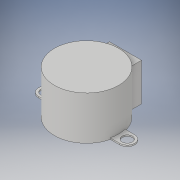
# Autodesk Inventor part: PasAPasCarcasse
Saved by Autodesk Inventor 2019 (Build 230136000, 136)
## iProperties
Created: 2020-12-11
Part Number: PasAPasCarcasse
Material: Générique
Document SubType Name: Modeling
Designer: tom.mousset
Density: 1 g/cm^3
Appearance: Par défaut
Author: tom.mousset
Autodesk Inventor part; units mm, degrees
ref_plane "YZ Plane" through (0, 0, 0) normal (1, 0, 0) x (0, 1, 0)
ref_plane "XZ Plane" through (0, 0, 0) normal (0, 1, 0) x (-1, 0, 0)
ref_plane "XY Plane" through (0, 0, 0) normal (0, 0, 1) x (1, 0, 0)
sketch "Esquisse1" plane through (0, 0, 0) normal (0, 1, 0) x (-1, 0, 0)
  circle A0 centre (0, 0) radius 14
  dimension "d0" = 28
  constraints: 1 centre point, 1 coincident
  measures "d0" diameter of A0
extrude "Extrusion1" add sketch "Esquisse1" along normal blind 19
sketch "Esquisse2" plane through (0, 0, 0) normal (0, -1, 0) x (1, 0, 0)
  line L0 (-21, -3.25) -> (21, -3.25)
  line L1 (21, -3.25) -> (21, 3.25)
  line L2 (21, 3.25) -> (-21, 3.25)
  line L3 (-21, 3.25) -> (-21, -3.25)
  line L4 (-21, -3.25) -> (21, 3.25) construction
  line L5 (21, -3.25) -> (-21, 3.25) construction
  circle A0 centre (-17.75, 0) radius 2.25
  circle A1 centre (17.75, 0) radius 2.25
  arc A2 (-17.75, 3.25) -> (-17.75, -3.25) centre (-17.75, 0) ccw
  arc A3 (17.75, -3.25) -> (17.75, 3.25) centre (17.75, 0) ccw
  circle A4 centre (0, 0) radius 14 projected
  arc A5 (13.6175, -3.25) -> (13.6175, 3.25) centre (0, 0) ccw
  arc A6 (-13.6175, 3.25) -> (-13.6175, -3.25) centre (0, 0) ccw
  line L6 (-17.75, 3.25) -> (-13.6175, 3.25)
  line L7 (-17.75, -3.25) -> (-13.6175, -3.25)
  line L8 (13.6175, -3.25) -> (17.75, -3.25)
  line L9 (17.75, 3.25) -> (13.6175, 3.25)
  dimension "d3" = 42
  dimension "d4" = 6.5
  dimension "d5" = 4.5
  dimension "d6" = 4.5
  dimension "d7" = 3.25
  dimension "d8" = 3.25
  constraints: 20 end point, 12 point on circle, 8 point on line, 6 centre point, 4 coincident, 4 collinear, 2 midpoint, 2 parallel, 1 horizontal, 1 perpendicular
  measures "d3" distance of L2.end L1.end
  measures "d4" distance of L1.end L0.end
  measures "d5" diameter of A0
  measures "d6" diameter of A1
  measures "d7" distance from line of L1 A1.centre
  measures "d8" distance from line of A0.centre L3
extrude "Extrusion2" add sketch "Esquisse2" against normal blind 0.6 contours A2 L2 A4 L0 | A4 L2 A3 L0
sketch "Esquisse3" plane through (0, 0, 0) normal (0, 0, 1) x (1, 0, 0)
  line L0 (7, 0) -> (-7, 0)
  line L1 (-7, 0) -> (-7, 16.5)
  line L2 (-7, 16.5) -> (7, 16.5)
  line L3 (7, 16.5) -> (7, 0)
  point P0 (0, 0)
  dimension "d11" = 16.5
  dimension "d14" = 14
  dimension "d15" = 7
  constraints: 8 end point, 2 parallel, 1 horizontal, 1 perpendicular
  measures "d11" distance of L0.end L1.end
  measures "d14" distance between parallel lines of L1 L3
  measures "d15" distance of point (0, 0) L0.start
extrude "Extrusion3" add sketch "Esquisse3" against normal blind 17
